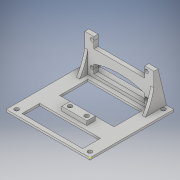
# Autodesk Inventor part: ProtoBoard
Saved by Autodesk Inventor 2019.1 (Build 231200000, 200)
## iProperties
Created: 2018-12-30
Part Number: ProtoBoard
Material: Generic
Document SubType Name: Modeling
Designer: acorbeau
Density: 1 g/cm^3
Appearance: Default
Author: acorbeau
Autodesk Inventor part; units mm, degrees
ref_plane "YZ Plane" through (0, 0, 0) normal (1, 0, 0) x (0, 1, 0)
ref_plane "XZ Plane" through (0, 0, 0) normal (0, 1, 0) x (-1, 0, 0)
ref_plane "XY Plane" through (0, 0, 0) normal (0, 0, 1) x (1, 0, 0)
sketch "Sketch1" plane through (0, 0, 0) normal (0, 1, 0) x (-1, 0, 0)
  line L0 (0, 0) -> (80, 0)
  line L1 (80, 0) -> (80, -80)
  line L2 (80, -80) -> (0, -80)
  line L3 (0, -80) -> (0, 0)
  line L4 (63.0847, -18.93) -> (13.0847, -18.93) construction
  line L5 (13.0847, -18.93) -> (13.0847, -23.93) construction
  line L6 (13.0847, -23.93) -> (63.0847, -23.93) construction
  line L7 (63.0847, -23.93) -> (63.0847, -18.93) construction
  line L8 (63.0847, -42.93) -> (13.0847, -42.93) construction
  line L9 (13.0847, -42.93) -> (13.0847, -47.93) construction
  line L10 (13.0847, -47.93) -> (63.0847, -47.93) construction
  line L11 (63.0847, -47.93) -> (63.0847, -42.93) construction
  line L12 (51.4414, -53.454) -> (27.4414, -53.454) construction
  line L13 (27.4414, -53.454) -> (27.4414, -61.454) construction
  line L14 (27.4414, -61.454) -> (51.4414, -61.454) construction
  line L15 (51.4414, -61.454) -> (51.4414, -53.454) construction
  circle A0 centre (48.4614, -57.454) radius 2 construction
  circle A1 centre (30.4614, -57.454) radius 2 construction
  dimension "d0" = 80
  dimension "d1" = 80
  dimension "d2" = 24
  dimension "d3" = 8
  dimension "d4" = 4
  dimension "d5" = 18
  dimension "d6" = 2.98
  dimension "d7" = 4
  dimension "d8" = 3.02
  dimension "d9" = 50
  dimension "d10" = 5
  dimension "d11" = 19
  constraints: 32 end point, 8 parallel, 4 horizontal, 4 perpendicular, 2 centre point, 2 point on line, 1 collinear, 1 equal radius
  measures "d0" distance of L0.end L1.end
  measures "d1" distance of L1.end L2.end
  measures "d2" distance of L12.start L12.end
  measures "d3" distance of L14.end L12.start
  measures "d4" diameter of A0
  measures "d5" distance of A1.centre A0.centre
  measures "d6" distance from line of L15 A0.centre
  measures "d7" distance from line of L12 A0.centre
  measures "d8" distance from line of L13 A1.centre
  measures "d9" distance of L9.end L10.end
  measures "d10" distance of L6.end L4.start
  measures "d11" distance between parallel lines of L6 L8
extrude "Extrusion1" add sketch "Sketch1" along normal blind 2
sketch "Sketch3" plane through (0, 2, 0) normal (0, 1, 0) x (1, 0, 0)
  circle A0 centre (-48.98, 29) radius 2 construction
  circle A1 centre (-30.98, 29) radius 2 construction
  line L0 (-28, 33) -> (-52, 33)
  line L1 (-52, 25) -> (-28, 25)
  line L2 (-28, 25) -> (-28, 33)
  line L3 (-52, 33) -> (-52, 25)
  line L4 (-80, 80) -> (-80, 0) construction
  line L5 (-80, 40) -> (0, 40) construction
  line L6 (0, 0) -> (0, 80) construction
  line L7 (0, 80) -> (-80, 80) construction
  line L8 (-40, 80) -> (-40, 0) construction
  line L9 (-80, 0) -> (0, 0) construction
  point P0 (-40, 33)
  dimension "d29" = 24
  dimension "d30" = 8
  dimension "d31" = 4
  dimension "d32" = 18
  dimension "d33" = 2.98
  dimension "d34" = 4
  dimension "d35" = 3.02
  dimension "d128" = 15
  constraints: 12 end point, 5 midpoint, 2 centre point, 2 parallel, 1 equal radius, 1 horizontal, 1 perpendicular, 1 point on line
  measures "d29" distance of L0.start L0.end
  measures "d30" distance of L1.end L0.start
  measures "d31" diameter of A1
  measures "d32" distance of A0.centre A1.centre
  measures "d33" distance from line of L2 A1.centre
  measures "d34" distance from line of L0 A1.centre
  measures "d35" distance from line of L3 A0.centre
  measures "d128" distance from line of L5 L1.start
extrude "Extrusion3" add sketch "Sketch3" along normal blind 4
sketch "Sketch4" plane through (0, 2, 0) normal (0, 1, 0) x (1, 0, 0)
  point P0 (0, 0)
sketch "Sketch7" plane through (0, 2, 0) normal (0, 1, 0) x (1, 0, 0)
  line L0 (-5, 5) -> (-75, 5)
  line L1 (-75, 5) -> (-75, 75)
  line L2 (-75, 75) -> (-5, 75)
  line L3 (-5, 75) -> (-5, 5)
  line L4 (-80, 0) -> (0, 0) projected
  line L5 (0, 0) -> (0, 80) projected
  line L6 (-80, 80) -> (-80, 0) projected
  line L7 (0, 80) -> (-80, 80) projected
  dimension "d49" = 5
  dimension "d50" = 5
  dimension "d51" = 5
  dimension "d52" = 5
  constraints: 8 end point, 4 coincident, 2 parallel, 1 horizontal, 1 perpendicular
  measures "d49" distance between parallel lines of L4 L0
  measures "d50" distance between parallel lines of L3 L5
  measures "d51" distance between parallel lines of L6 L1
  measures "d52" distance between parallel lines of L7 L2
hole "Hole2" at (-5, 2, -5) at (-5, 2, -75) at (-75, 2, -75) at (-75, 2, -5) direction (0, -1, 0) diameter 4 end through all
sketch "Sketch10" plane through (0, 6, 0) normal (0, 1, 0) x (1, 0, 0)
  line L0 (-52, 33) -> (-52, 25) projected
  line L1 (-52, 29) -> (-29.1848, 29)
  point P0 (0, 0)
  point P1 (-48.1206, 29)
  point P2 (-32.1206, 29)
  dimension "d81" = 16
  constraints: 2 end point, 2 point on line, 1 horizontal, 1 midpoint
  measures "d81" distance of point (-32.121, 29) point (-48.121, 29)
hole "Hole3" at (-48.1206, 6, -29) at (-32.1206, 6, -29) direction (0, -1, 0) diameter 4 end through all
sketch "Sketch20" plane through (0, 2, 0) normal (0, 1, 0) x (1, 0, 0)
  line L0 (-73, 80) -> (-70, 80) construction
  line L1 (-70, 60) -> (-73, 60) construction
  line L2 (-73, 60) -> (-73, 80) construction
  line L3 (-10, 60) -> (-7, 60) construction
  line L4 (-7, 60) -> (-7, 80) construction
  line L5 (-7, 80) -> (-10, 80) construction
  line L6 (-70, 60) -> (-73, 60)
  line L7 (-73, 60) -> (-73, 80)
  line L8 (-73, 80) -> (-70, 80)
  line L9 (-70, 80) -> (-70, 72)
  line L10 (-70, 72) -> (-10, 72)
  line L11 (-10, 72) -> (-10, 80)
  line L12 (-10, 80) -> (-7, 80)
  line L13 (-7, 80) -> (-7, 60)
  line L14 (-7, 60) -> (-10, 60)
  line L15 (-10, 60) -> (-10, 68)
  line L16 (-10, 68) -> (-70, 68)
  line L17 (-70, 68) -> (-70, 60)
  line L18 (-70, 60) -> (-73, 60)
  point P0 (0, 0)
  dimension "d132" = 3
  dimension "d133" = 20
  constraints: 38 end point, 7 perpendicular, 3 equal length, 2 horizontal, 1 collinear, 1 point on line
  measures "d132" distance of L0.start L0.end
  measures "d133" distance of L1.end L0.start
extrude "Extrusion13" add sketch "Sketch20" along normal blind 34
sketch "Sketch21" plane through (-70, 2, -60) normal (1, 0, 0) x (0, 0, -1)
  line L0 (8, 0) -> (0, 0) construction
  line L1 (0, 0) -> (5.8768, 9.0116) construction
  line L2 (8, 0) -> (8, 34) construction
  line L3 (5.8768, 9.0116) -> (8, 20.3813) construction
  spline S0 degree 2 poles (0, 0) (5.8768, 9.0116) (8, 20.3813) knots 1 1 1 2 2 2
  line L4 (0, 0) -> (0, 34) projected
  line L5 (0, 0) -> (0, 34)
  line L6 (0, 34) -> (8, 34) projected
  line L7 (0, 34) -> (8, 34)
  line L8 (8, 34) -> (8, 20.3813)
  point P0 (-60, -2)
  constraints: 6 end point, 1 collinear, 1 perpendicular, 1 point on line, 1 vertical, 3 other
extrude "Extrusion14" cut sketch "Sketch21" along normal through all both and the other way through all
sketch "Sketch22" plane through (-70, 2, -72) normal (1, 0, 0) x (0, 0, -1)
  line L0 (0, 34) -> (8, 0)
  line L1 (8, 0) -> (8, 34)
  line L2 (0, 34) -> (8, 34) projected
  line L3 (8, 34) -> (0, 34)
  point P0 (-72, -2)
  constraints: 6 end point
extrude "Extrusion15" cut sketch "Sketch22" along normal through all both and the other way through all
sketch "Sketch23" plane through (-70, 2, -68) normal (0, 0, 1) x (1, 0, 0)
  line L0 (4, 7.5) -> (56, 7.5)
  line L1 (56, 7.5) -> (56, 30.5)
  line L2 (56, 30.5) -> (4, 30.5)
  line L3 (4, 30.5) -> (4, 7.5)
  line L4 (4, 7.5) -> (56, 30.5)
  line L5 (56, 7.5) -> (4, 30.5)
  line L6 (30, 30.5) -> (30, 34) construction
  line L7 (-3, 34) -> (63, 34) construction
  line L8 (30, 7.5) -> (30, 4) construction
  line L9 (18, 4) -> (42, 4) projected
  point P0 (70, -2)
  point P1 (30, 19)
  dimension "d142" = 52
  dimension "d143" = 23
  constraints: 16 end point, 6 midpoint, 2 parallel, 1 collinear, 1 horizontal, 1 perpendicular, 1 vertical
  measures "d142" distance of L1.end L2.end
  measures "d143" distance of L2.end L0.start
hole "Hole5" at (-14, 32.5, -68) at (-14, 9.5, -68) at (-66, 9.5, -68) at (-66, 32.5, -68) direction (0, 0, -1) diameter 3.5 end through all
sketch "Sketch24" plane through (-70, 2, -68) normal (0, 0, 1) x (1, 0, 0)
  line L0 (60, 34) -> (0, 34) construction
  line L1 (5.75, 34) -> (54.25, 34)
  line L2 (54.25, 34) -> (54.25, 24)
  line L3 (54.25, 24) -> (5.75, 24)
  line L4 (5.75, 24) -> (5.75, 34)
  circle A0 centre (4, 30.5) radius 1.75 construction
  circle A1 centre (56, 30.5) radius 1.75 construction
  point P0 (70, -2)
  dimension "d151" = 0
  dimension "d152" = 0
  dimension "d153" = 10
  constraints: 8 end point, 2 parallel, 1 horizontal, 1 perpendicular, 1 point on line
  measures "d151" distance edge to line of A0 L4
  measures "d152" distance edge to line of A1 L2
  measures "d153" distance of L3.end L1.start
extrude "Extrusion16" cut sketch "Sketch24" against normal blind 34
sketch "Sketch25" plane through (-70, 2, -68) normal (0, 0, 1) x (1, 0, 0)
  line L0 (5.75, 3) -> (54.25, 3)
  line L1 (54.25, 3) -> (54.25, 11.4232)
  line L2 (54.25, 11.4232) -> (5.75, 11.4232) construction
  line L3 (5.75, 11.4232) -> (5.75, 3)
  line L4 (60, 0) -> (0, 0) construction
  circle A0 centre (4, 7.5) radius 1.75 construction
  circle A1 centre (56, 7.5) radius 1.75 construction
  arc A2 (54.25, 11.4232) -> (5.75, 11.4232) centre (30, -60.0846) ccw
  line L5 (30, 15.4232) -> (30, 11.4232) construction
  point P0 (70, -2)
  dimension "d156" = 3
  dimension "d157" = 8.4232
  dimension "d159" = 0
  dimension "d160" = 0
  dimension "d161" = 4
  constraints: 10 end point, 3 point on circle, 2 parallel, 1 centre point, 1 horizontal, 1 midpoint, 1 perpendicular
  measures "d156" distance between parallel lines of L0 L4
  measures "d157" distance of L2.end L0.start
  measures "d159" distance edge to line of A0 L3
  measures "d160" distance edge to line of A1 L1
  measures "d161" distance of L5.start L5.end
extrude "Extrusion17" cut sketch "Sketch25" against normal blind 34
sketch "Sketch26" plane through (0, 2, 0) normal (0, 1, 0) x (1, 0, 0)
  line L0 (-66, 64) -> (-14, 64)
  line L1 (-14, 64) -> (-14, 37)
  line L2 (-14, 37) -> (-66, 37)
  line L3 (-66, 37) -> (-66, 64)
  line L4 (-70, 68) -> (-70, 60) construction
  line L5 (-10, 60) -> (-10, 68) projected
  line L6 (-15.75, 68) -> (-64.25, 68) construction
  line L7 (-28, 33) -> (-52, 33) projected
  line L8 (-80, 0) -> (0, 0) construction
  dimension "d164" = 4
  dimension "d165" = 4
  dimension "d166" = 4
  dimension "d167" = 4
  constraints: 8 end point, 2 parallel, 1 horizontal, 1 perpendicular
  measures "d164" distance between parallel lines of L4 L3
  measures "d165" distance between parallel lines of L1 L5
  measures "d166" distance between parallel lines of L0 L6
  measures "d167" distance between parallel lines of L2 L7
extrude "Extrusion18" cut sketch "Sketch26" against normal blind 34
sketch "Sketch27" plane through (0, 2, 0) normal (0, 1, 0) x (1, 0, 0)
  line L0 (-69, 21) -> (-11, 21)
  line L1 (-11, 21) -> (-11, 4)
  line L2 (-11, 4) -> (-69, 4)
  line L3 (-69, 4) -> (-69, 21)
  line L4 (-52, 25) -> (-28, 25) construction
  line L5 (-80, 0) -> (0, 0) construction
  circle A0 centre (-75, 5) radius 2 construction
  circle A1 centre (-5, 5) radius 2 construction
  dimension "d172" = 4
  dimension "d173" = 4
  dimension "d174" = 4
  dimension "d175" = 4
  constraints: 8 end point, 2 parallel, 1 horizontal, 1 perpendicular
  measures "d172" distance between parallel lines of L4 L0
  measures "d173" distance between parallel lines of L5 L2
  measures "d174" distance edge to line of A0 L3
  measures "d175" distance edge to line of A1 L1
extrude "Extrusion19" cut sketch "Sketch27" against normal blind 34
body "Solid1"
